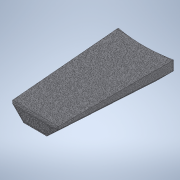
# Autodesk Inventor part: Surtidor
Saved by Autodesk Inventor 2020 (Build 240168000, 168)
## iProperties
Created: 2020-10-28
Part Number: Surtidor
Material: Iron, Cast
Document SubType Name: Modeling
Designer: aaron
Density: 7.15 g/cm^3
Appearance: Iron - Cast
Author: aaron
## iProperties of the stored document _3DPrint.ipt
Created: 2020-11-03
Part Number: _3DPrint
Material: Generic
Document SubType Name: Modeling
Designer: aaron
Density: 1 g/cm^3
Appearance: Default
Author: aaron
Autodesk Inventor part; units mm, degrees
ref_plane "YZ Plane" through (0, 0, 0) normal (1, 0, 0) x (0, 1, 0)
ref_plane "XZ Plane" through (0, 0, 0) normal (0, 1, 0) x (-1, 0, 0)
sketch "Sketch1" plane through (0, 0, 0) normal (0, 0, 1) x (1, 0, 0)
  line L0 (0, 0) -> (17.5, 0)
  line L1 (17.5, 0) -> (17.5, -6)
  line L2 (17.5, -6) -> (8.5, -15)
  line L3 (8.5, -15) -> (0, -15)
  line L4 (0, 0) -> (0, -15)
  line L5 (0, 0) -> (-17.5, 0)
  line L6 (-17.5, 0) -> (-17.5, -6)
  line L7 (-17.5, -6) -> (-8.5, -15)
  line L8 (-8.5, -15) -> (0, -15)
  dimension "d0" = 35
  dimension "d1" = 15
  dimension "d2" = 45
  dimension "d3" = 6
  constraints: 18 end point, 3 symmetric about line, 2 perpendicular, 1 horizontal, 1 parallel
  measures "d0" diameter of L1 L4
  measures "d1" distance between parallel lines of L3 L0
  measures "d2" angle of L3 L2
  measures "d3" distance of L0.end L1.end
ref_plane "Work Plane1" through (0, 0, 70) normal (0, 0, 1) x (1, 0, 0)
sketch "Sketch2" plane through (0, 0, 70) normal (0, 0, 1) x (1, 0, 0)
  line L0 (-17.5, -6) -> (-8.5, -15) projected
  line L1 (-17.5, 0) -> (-17.5, -6) projected
  line L2 (0, 0) -> (-17.5, 0) projected
  line L3 (0, 0) -> (17.5, 0) projected
  line L4 (17.5, 0) -> (17.5, -6) projected
  line L5 (17.5, -6) -> (8.5, -15) projected
  line L6 (8.5, -15) -> (0, -15) projected
  line L7 (-8.5, -15) -> (0, -15) projected
  line L8 (-14.5, -4.7574) -> (-7.2574, -12)
  line L9 (-7.2574, -12) -> (0, -12)
  line L10 (0, -12) -> (7.2574, -12)
  line L11 (7.2574, -12) -> (14.5, -4.7574)
  line L12 (14.5, -4.7574) -> (14.5, -3)
  line L13 (14.5, -3) -> (0, -3)
  line L14 (0, -3) -> (-14.5, -3)
  line L15 (-14.5, -3) -> (-14.5, -4.7574)
  dimension "d5" = 3
  constraints: 16 end point, 7 other
  measures "d5" distance between parallel lines of L1 L15
extrude "Extrusion1" add sketch "Sketch1" along normal blind 1
extrude "Extrusion2" add sketch "Sketch2" along normal blind 1 contours L15 L14 L13 L12 L11 L10 L9 L8
loft "Loft1" add section 1 edges at (-13, -10.5, 1) (0, -15, 1) (13, -10.5, 1) (17.5, -3, 1) (0, 0, 1) (-17.5, -3, 1) section 2 edges at (0, -3, 70) (14.5, -3.8787, 70) (10.8787, -8.3787, 70) (0, -12, 70) (-10.8787, -8.3787, 70) (-14.5, -3.8787, 70)
sketch "Sketch6" plane through (0, 0, 0) normal (1, 0, 0) x (0, 1, 0)
  line L0 (-15, 1) -> (-12, 70) projected
  line L1 (-12, 70) -> (-12, 71) projected
  line L2 (-12, 71) -> (-3, 71) projected
  line L3 (-3, 71) -> (-3, 70) projected
  line L4 (-3, 70) -> (0, 1) projected
  line L5 (0, 1) -> (0, 0) projected
  line L6 (0, 0) -> (-15, 0) projected
  line L7 (-15, 0) -> (-15, 1) projected
  line L8 (-6, 0) -> (-15, 0) projected
  line L9 (-7.5, 0) -> (-7.5, 61)
  line L10 (-11.5, 65) -> (-15, 65)
  arc A0 (-7.5, 61) -> (-11.5, 65) centre (-11.5, 61) ccw
  point P0 (-7.5, 65)
  dimension "d20" = 65
  dimension "d21" = 4
  dimension "d23" = 7.5
  dimension "d24" = 15
  constraints: 4 end point, 3 point on line, 2 perpendicular, 2 point on circle, 2 tangent, 1 centre point
  measures "d20" distance of L9.start point (-7.5, 65)
  measures "d21" radius of A0
  measures "d23" distance between parallel lines of L5 L9
  measures "d24" distance from line of L10.end L5
sketch "Sketch7" plane through (0, 0, 0) normal (0, 0, -1) x (-1, 0, 0)
  line L0 (17.5, 0) -> (17.5, -6) projected
  line L1 (17.5, -6) -> (8.5, -15) projected
  line L2 (8.5, -15) -> (-8.5, -15) projected
  line L3 (-8.5, -15) -> (-17.5, -6) projected
  line L4 (-17.5, -6) -> (-17.5, 0) projected
  line L5 (-17.5, 0) -> (17.5, 0) projected
  line L6 (17.5, -6) -> (8.5, -15) projected
  line L7 (17.5, 0) -> (17.5, -6) projected
  line L8 (-17.5, 0) -> (17.5, 0) projected
  line L9 (-17.5, -6) -> (-17.5, 0) projected
  line L10 (-8.5, -15) -> (-17.5, -6) projected
  line L11 (8.5, -15) -> (-8.5, -15) projected
  circle A0 centre (0, -7.5) radius 1.5
  point P0 (0, 0)
  dimension "d25" = 7.5
  dimension "d26" = 3
  dimension "d27" = 17.5
  constraints: 1 centre point
  measures "d25" distance from line of L5 A0.centre
  measures "d26" diameter of A0
  measures "d27" distance from line of A0.centre L0
sweep "Sweep1" cut profiles "Sketch7" path "Sketch6" path curves L9 A0 L10 contours A0
sketch "Sketch8" plane through (0, 0, 0) normal (0, 0, -1) x (-1, 0, 0)
  circle A0 centre (0, -7.5) radius 1.5 projected
  line L0 (17.5, -6) -> (8.5, -15) projected
  line L1 (17.5, 0) -> (17.5, -6) projected
  line L2 (-17.5, 0) -> (17.5, 0) projected
  line L3 (-17.5, -6) -> (-17.5, 0) projected
  line L4 (-8.5, -15) -> (-17.5, -6) projected
  line L5 (8.5, -15) -> (-8.5, -15) projected
  circle A1 centre (0, -7.5) radius 4.5
  point P0 (0, 0)
  dimension "d30" = 9
  constraints: 1 centre point, 1 coincident
  measures "d30" diameter of A1
extrude "Extrusion4" cut sketch "Sketch8" against normal blind 5 contours A1
fillet "Fillet1" radius 0.5 1 edges at (4.5, -7.5, 0)
fillet "Fillet2" radius 2 6 edges at (10.8787, -8.3787, 71) (0, -12, 71) (-10.8787, -8.3787, 71) (-14.5, -3.8787, 71) (0, -3, 71) (14.5, -3.8787, 71)
sketch "Sketch9" plane through (-17.5, 0, 1) normal (0, 0.9990562, 0.0434372) x (1, 0, 0)
  line L0 (0, 0.9991) -> (0, 0) projected
  line L1 (35, 0.9991) -> (0, 0.9991) projected
  line L2 (35, 0.9991) -> (35, 0) projected
  arc A0 (0, 0.9991) -> (35, 0.9991) centre (17.5, 89.2813) ccw
  point P0 (17.5, 0.9991)
  dimension "d35" = 90
  constraints: 2 point on circle, 1 centre point
  measures "d35" radius of A0
extrude "Extrusion5" cut sketch "Sketch9" against normal through all
body "Solid1"
